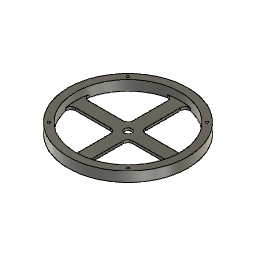
main_body_48mm_diameter v1 (Autodesk Fusion 360 design; units mm, degrees)
Autodesk Fusion 360 part; units mm, degrees
sketch "Sketch1" plane through (0, 0, 0) normal (0, 0, 1) x (1, 0, 0)
  circle A0 centre (0, 0) radius 24
  circle A1 centre (0, 0) radius 21
  line L0 (-2.5, 4.5) -> (-2.5, 18.4793)
  line L1 (2.5, 18.4793) -> (2.5, 4.5)
  line L2 (4.5, 2.5) -> (18.4795, 2.5)
  line L3 (18.4604, -2.5) -> (4.5, -2.5)
  line L4 (-2.5, -4.5) -> (-2.5, -18.4675)
  line L5 (2.5, -18.4675) -> (2.5, -4.5)
  line L6 (-4.5, 2.5) -> (-18.4663, 2.5)
  line L7 (-18.4663, -2.5) -> (-4.5, -2.5)
  arc A2 (2.5, 4.5) -> (4.5, 2.5) centre (4.5, 4.5) ccw
  arc A3 (4.5, -2.5) -> (2.5, -4.5) centre (4.5, -4.5) ccw
  arc A4 (-2.5, -4.5) -> (-4.5, -2.5) centre (-4.5, -4.5) ccw
  arc A5 (-4.5, 2.5) -> (-2.5, 4.5) centre (-4.5, 4.5) ccw
  line L8 (4.8374, 20.4506) -> (4.5763, 20.4953)
  line L9 (-4.8374, 20.4506) -> (-4.5763, 20.4953)
  arc A6 (-2.5, 18.4793) -> (-4.8374, 20.4506) centre (-4.5, 18.4793) ccw
  arc A7 (4.8374, 20.4506) -> (2.5, 18.4793) centre (4.5, 18.4793) ccw
  line L10 (20.4509, 4.8372) -> (20.4962, 4.5723)
  line L11 (20.4291, -4.8528) -> (20.4213, -4.8958)
  arc A8 (20.4291, -4.8528) -> (18.4604, -2.5) centre (18.4604, -4.5) ccw
  arc A9 (18.4795, 2.5) -> (20.4509, 4.8372) centre (18.4795, 4.5) ccw
  line L12 (4.847, -20.4372) -> (4.7758, -20.4497)
  line L13 (-4.847, -20.4372) -> (-4.7758, -20.4497)
  arc A10 (-4.847, -20.4372) -> (-2.5, -18.4675) centre (-4.5, -18.4675) ccw
  arc A11 (2.5, -18.4675) -> (4.847, -20.4372) centre (4.5, -18.4675) ccw
  line L14 (-20.4358, 4.848) -> (-20.4448, 4.797)
  line L15 (-20.4358, -4.848) -> (-20.4448, -4.797)
  arc A12 (-18.4663, -2.5) -> (-20.4358, -4.848) centre (-18.4663, -4.5) ccw
  arc A13 (-20.4358, 4.848) -> (-18.4663, 2.5) centre (-18.4663, 4.5) ccw
  circle A14 centre (0, 0) radius 1.5
  dimension "d1" = 48
  dimension "d2" = 42
  dimension "d6" = 2
  dimension "d7" = 2
  dimension "d8" = 2
  dimension "d9" = 2
  dimension "d10" = 2
  dimension "d11" = 2
  dimension "d12" = 2
  dimension "d13" = 2
  dimension "d14" = 2
  dimension "d15" = 2
  dimension "d16" = 2
  dimension "d17" = 2
  dimension "d18" = 3
  constraint concentric A0 A1
  constraint vertical L0
  constraint vertical L1
  constraint horizontal L2
  constraint horizontal L3
  constraint vertical L4
  constraint vertical L5
  constraint horizontal L6
  constraint horizontal L7
  constraint tangent L1 A2
  constraint tangent L2 A2
  constraint tangent L3 A3
  constraint tangent L5 A3
  constraint tangent L7 A4
  constraint tangent L4 A4
  constraint tangent L6 A5
  constraint tangent L0 A5
  constraint coincident A1 L8.end
  constraint coincident A1 L9.end
  constraint tangent L9 A6
  constraint tangent L0 A6
  constraint tangent L8 A7
  constraint tangent L1 A7
  constraint coincident A1 L10.end
  constraint coincident A1 L11.end
  constraint tangent L3 A8
  constraint tangent L11 A8
  constraint tangent L2 A9
  constraint tangent L10 A9
  constraint coincident A1 L12.end
  constraint coincident A1 L13.end
  constraint tangent L13 A10
  constraint tangent L4 A10
  constraint tangent L12 A11
  constraint tangent L5 A11
  constraint coincident A1 L14.end
  constraint coincident A1 L15.end
  constraint tangent L7 A12
  constraint tangent L15 A12
  constraint tangent L14 A13
  constraint tangent L6 A13
  constraint concentric A0 A14
  measures "d1" diameter of A0
  measures "d2" diameter of A1
  measures "d6" radius of A2
  measures "d7" radius of A3
  measures "d8" radius of A4
  measures "d9" radius of A5
  measures "d10" radius of A6
  measures "d11" radius of A7
  measures "d12" radius of A8
  measures "d13" radius of A9
  measures "d14" radius of A10
  measures "d15" radius of A11
  measures "d16" radius of A12
  measures "d17" radius of A13
  measures "d18" diameter of A14
extrude "Extrude1" add sketch "Sketch1" along normal blind 1 contours A1 L0 L1 L2 L3 L4 L5 L6 L7 A2 A3 A4 A5 A6 A7 L11 A8 A9 A10 A11 A12 A13
sketch "Sketch2" plane through (0, 0, 0) normal (0, 0, 1) x (1, 0, 0)
  circle A0 centre (0, 0) radius 21
  circle A1 centre (0, 0) radius 24
  line L0 (0, 0) -> (21, 0) construction
  line L1 (0, 0) -> (22.5, 0) construction
  circle A2 centre (15.9099, 15.9099) radius 0.5
  circle A3 centre (15.9099, -15.9099) radius 0.5
  circle A4 centre (-15.9099, -15.9099) radius 0.5
  circle A5 centre (-15.9099, 15.9099) radius 0.5
  dimension "d21" = 42
  dimension "d22" = 48
  dimension "d26" = 1
  dimension "d27" = 1
  dimension "d28" = 1
  dimension "d29" = 1
  constraint coincident A0.centre A1.centre
  constraint horizontal L0
  constraint horizontal L1
  constraint coincident A0 L0.end
  measures "d21" diameter of A0
  measures "d22" diameter of A1
  measures "d26" diameter of A2
  measures "d27" diameter of A3
  measures "d28" diameter of A4
  measures "d29" diameter of A5
extrude "Extrude2" add sketch "Sketch2" along normal blind 4
